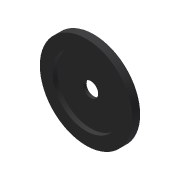
# Autodesk Inventor part: top plate washer
Saved by Autodesk Inventor 2022 Beta2 (Build 260130000, 130) ContinuousBuild 0
## iProperties
Shininess: 64.0
Length Units: 11272
Angle Units: 11279
Time Units: 11290
Mass Units: 11286
Length Display Precision: 3
Angle Display Precision: 2
Compacted: True
Part Number: top plate washer
Document SubType Name: Modeling
Created: 2003-04-07
Designer: demo
Density: 1 g/cm^3
Material: Generic
Appearance: Generic
Density: 0.0
Volumn: 0.0
Area: 0.0
PropertySet Name: Model Information
Control State: 0
Master: False
Checked Out: False
Author: demo
Autodesk Inventor part; units mm, degrees
ref_plane "YZ Plane" through (0, 0, 0) normal (1, 0, 0) x (0, 1, 0)
ref_plane "XZ Plane" through (0, 0, 0) normal (0, 1, 0) x (-1, 0, 0)
ref_plane "XY Plane" through (0, 0, 0) normal (0, 0, 1) x (1, 0, 0)
sketch "Sketch1" plane through (0, 0, 0) normal (0, 0, 1) x (1, 0, 0)
  circle A0 centre (-29.7426, 29.7426) radius 3.2004 projected
  circle A1 centre (29.7426, -29.7426) radius 3.2004 projected
  circle A2 centre (0, 0) radius 8.001 projected
  circle A3 centre (0, 0) radius 50.1904 projected
extrude "Extrusion1" add sketch "Sketch1" along normal blind 8.3312 contours A0 | A1 | A2 | A3
sketch "Sketch2" plane through (0, 0, 8.3312) normal (0, 0, 1) x (1, 0, 0)
  circle A0 centre (0, 0) radius 50.1904 projected
  circle A1 centre (0, 0) radius 36.4998
  dimension "d2" = 72.9996
  constraints: 1 centre point, 1 coincident, 1 concentric
  measures "d2" diameter of A1
extrude "Extrusion2" cut sketch "Sketch2" against normal blind 5.0038 contours A1
sketch "Sketch3" plane through (0, 0, 3.3274) normal (0, 0, 1) x (1, 0, 0)
  circle A0 centre (0, 0) radius 36.4998 projected
  circle A1 centre (0, 0) radius 8.001
  dimension "d5" = 16.002
  constraints: 1 centre point, 1 coincident, 1 concentric
  measures "d5" diameter of A1
extrude "Extrusion3" cut sketch "Sketch3" against normal through all contours A1
body "Solid1"
